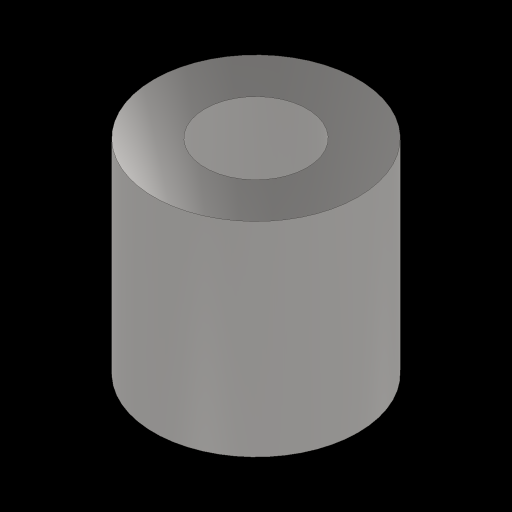
# Autodesk Inventor part: 4 x 8 x 8 mm Needle Bearing Mockup
Saved by Autodesk Inventor 2023 (Build 270158000, 158)
## iProperties
Created: 2023-08-01
Part Number: 4 x 8 x 8 mm Needle Bearing Mockup
Material: Stainless Steel
Document SubType Name: Modeling
Designer: tandu
Density: 6.63146 g/cm^3
Appearance: Semi-Polished
Mass: 2 g
Surface Area: 3.76991 cm^2
Volume: 0.301593 cm^3
Author: tandu
Autodesk Inventor part; units mm, degrees
ref_plane "YZ Plane" through (0, 0, 0) normal (1, 0, 0) x (0, 1, 0)
ref_plane "XZ Plane" through (0, 0, 0) normal (0, 1, 0) x (-1, 0, 0)
ref_plane "XY Plane" through (0, 0, 0) normal (0, 0, 1) x (1, 0, 0)
sketch "Sketch1" plane through (0, 0, 0) normal (0, 1, 0) x (-1, 0, 0)
  circle A0 centre (0, 0) radius 2
  circle A1 centre (0, 0) radius 4
  dimension "d0" = 4
  dimension "d1" = 8
  constraints: 2 centre point, 2 coincident
  measures "d0" diameter of A0
  measures "d1" diameter of A1
extrude "Extrusion1" add sketch "Sketch1" along normal mid plane 8
body "Solid1"
